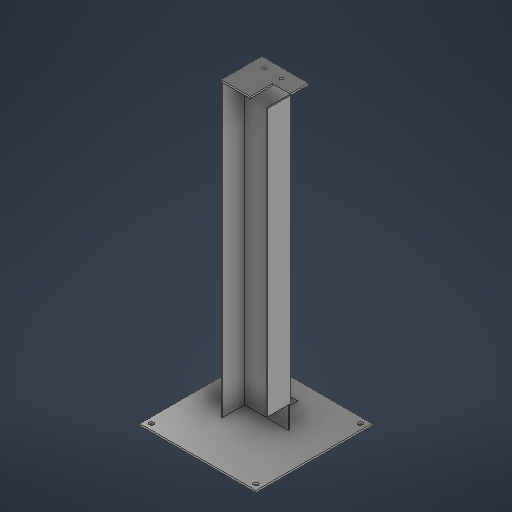
# Autodesk Inventor part: Poste
Saved by Autodesk Inventor 2026 (Build 300175050, 175E)
## iProperties
Created: 2025-07-17
Part Number: Poste
Material: Acero, carbono
Document SubType Name: Modeling
Designer: bello
Density: 7.85 g/cm^3
Appearance: Semipulido
Author: bello
Autodesk Inventor part; units mm, degrees
ref_plane "YZ Plane" through (0, 0, 0) normal (1, 0, 0) x (0, 1, 0)
ref_plane "XZ Plane" through (0, 0, 0) normal (0, 1, 0) x (-1, 0, 0)
ref_plane "XY Plane" through (0, 0, 0) normal (0, 0, 1) x (1, 0, 0)
sketch "Boceto1" plane through (0, 0, 0) normal (0, 1, 0) x (-1, 0, 0)
  line L0 (-100, 100) -> (100, 100)
  line L1 (100, 100) -> (100, -100)
  line L2 (100, -100) -> (-100, -100)
  line L3 (-100, -100) -> (-100, 100)
  line L4 (-100, 100) -> (100, -100) construction
  line L5 (100, 100) -> (-100, -100) construction
  point P0 (0, 0)
  dimension "d0" = 200
  dimension "d1" = 200
  constraints: 12 end point, 2 midpoint, 2 parallel, 1 horizontal, 1 perpendicular
  measures "d0" distance of L0.end L1.end
  measures "d1" distance of L1.end L2.end
extrude "Extrusión1" add sketch "Boceto1" along normal blind 3
sketch "Boceto2" plane through (0, 3, 0) normal (0, 1, 0) x (1, 0, 0)
  circle A0 centre (90, 90) radius 4
  line L0 (100, 100) -> (-100, 100) projected
  line L1 (100, -100) -> (100, 100) projected
  line L2 (0, 183.7429) -> (0, -123.1755)
  line L3 (-226.0201, 0) -> (210.3081, 0)
  circle A1 centre (-90, 90) radius 4
  circle A2 centre (90, -90) radius 4
  circle A3 centre (-90, -90) radius 4
  point P0 (0, 0)
  dimension "d4" = 8
  dimension "d5" = 10
  dimension "d6" = 10
  constraints: 4 centre point, 4 end point, 3 symmetric about line, 1 horizontal, 1 vertical, 3 other
  measures "d4" diameter of A0
  measures "d5" distance from line of L0 A0.centre
  measures "d6" distance from line of L1 A0.centre
hole "Agujero1" at (-90, 3, -90) at (90, 3, -90) at (-90, 3, 90) at (90, 3, 90) direction (0, -1, 0) diameter 8 end through all
sketch "Boceto3" plane through (0, 3, 0) normal (0, 1, 0) x (1, 0, 0)
  line L0 (-38, -20) -> (-38, 18)
  line L1 (-38, 18) -> (0, 18)
  line L2 (0, 18) -> (38, 18)
  line L3 (38, 18) -> (38, -20)
  line L4 (38, -20) -> (40, -20)
  line L5 (40, -20) -> (40, 20)
  line L6 (40, 20) -> (-40, 20)
  line L7 (-40, 20) -> (-40, -20)
  line L8 (-40, -20) -> (-38, -20)
  point P0 (0, 0)
  dimension "d14" = 40
  dimension "d15" = 80
  dimension "d16" = 2
  dimension "d17" = 38
  dimension "d18" = 40
  dimension "d19" = 20
  constraints: 18 end point, 7 perpendicular, 2 collinear, 2 point on line, 1 vertical
  measures "d14" distance of L6.end L7.end
  measures "d15" distance of L5.end L6.end
  measures "d16" distance of L3.end L4.end
  measures "d17" distance of L2.end L3.end
  measures "d18" distance from line of L7 point (0, 0)
  measures "d19" distance from line of point (0, 0) L6
extrude "Extrusión2" add sketch "Boceto3" along normal blind 500
ref_plane "Plano de trabajo1" through (0, 3, -18) normal (-1, 0, 0) x (0, 0, 1)
sketch "Boceto5" plane through (0, 3, -18) normal (-1, 0, 0) x (0, 0, 1)
  line L0 (-52, 0) -> (-2, 50)
  line L1 (-82, -3) -> (118, -3) projected
  point P0 (18, -3)
  point P1 (-2, 0)
  dimension "d26" = 50
  constraints: 2 end point
  measures "d26" distance of point (-2, 0) L0.start
extrude "Nervio1" add sketch "Boceto5" along normal mid plane 5 rib yes fills toward (-26.9646, 24.9646) open curves L0
sketch "Boceto6" plane through (40, 3, 20) normal (1, 0, 0) x (0, 0, -1)
  line L0 (40, 0) -> (40, 500) projected
  line L1 (40, 0) -> (40, 40)
  line L2 (40, 40) -> (0, 40)
  line L3 (0, 0) -> (0, 500) projected
  line L4 (0, 40) -> (0, 0)
  line L5 (0, 0) -> (40, 0)
  point P0 (20, -3)
  constraints: 8 end point, 2 point on line, 1 horizontal, 1 perpendicular, 1 vertical
extrude "Extrusión3" cut sketch "Boceto6" against normal blind 2
sketch "Boceto7" plane through (-38, 3, -18) normal (0, 0, 1) x (1, 0, 0)
  circle A0 centre (58, 30) radius 4
  line L0 (78, 40) -> (78, 500) projected
  point P0 (38, -3)
  dimension "d37" = 8
  dimension "d52" = 20
  constraints: 1 centre point
  measures "d37" diameter of A0
  measures "d52" distance from line of A0.centre L0
extrude "Extrusión4" cut sketch "Boceto7" against normal blind 5
sketch "Boceto10" plane through (0, 503, 0) normal (0, 1, 0) x (1, 0, 0)
  line L0 (-38, -20) -> (-40, -20) projected
  line L1 (-40, -20) -> (-40, 50)
  line L2 (-40, 50) -> (40, 50)
  line L3 (40, 50) -> (40, 18)
  line L4 (40, 18) -> (10, 18)
  line L5 (2.5, 20) -> (38, 20) projected
  line L6 (10, 18) -> (10, -20)
  line L7 (10, -20) -> (-40, -20)
  point P0 (0, 0)
  dimension "d58" = 70
  dimension "d59" = 50
  dimension "d60" = 30
  constraints: 12 end point, 3 perpendicular, 1 horizontal, 1 parallel, 1 vertical
  measures "d58" distance of L0.end L1.end
  measures "d59" distance of L6.end L0.end
  measures "d60" distance of L3.end L4.end
extrude "Extrusión7" add sketch "Boceto10" along normal blind 3
sketch "Boceto11" plane through (0, 506, 0) normal (0, 1, 0) x (1, 0, 0)
  circle A0 centre (-20, 34) radius 3
  circle A1 centre (10, 34) radius 3
  line L0 (40, 50) -> (-40, 50) projected
  line L1 (-40, 50) -> (-40, -20) projected
  line L2 (40, 18) -> (40, 50) projected
  point P0 (0, 0)
  dimension "d63" = 16
  dimension "d64" = 16
  dimension "d65" = 6
  dimension "d67" = 30
  dimension "d70" = 30
  constraints: 2 centre point, 1 equal radius
  measures "d63" distance from line of L0 A0.centre
  measures "d64" distance from line of L0 A1.centre
  measures "d65" diameter of A0
  measures "d67" distance from line of L2 A1.centre
  measures "d70" distance of A0.centre A1.centre
extrude "Extrusión8" cut sketch "Boceto11" against normal blind 3
